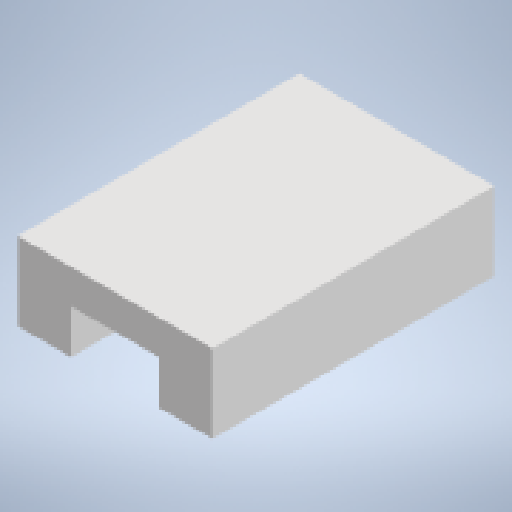
# Autodesk Inventor part: Carrige
Saved by Autodesk Inventor 2023 (Build 270158000, 158)
## iProperties
Created: 2022-09-16
Part Number: Carrige
Material: Generic
Document SubType Name: Modeling
Designer: deli
Density: 1 g/cm^3
Appearance: Default
Author: deli
Autodesk Inventor part; units mm, degrees
ref_plane "YZ Plane" through (0, 0, 0) normal (1, 0, 0) x (0, 1, 0)
ref_plane "XZ Plane" through (0, 0, 0) normal (0, 1, 0) x (-1, 0, 0)
ref_plane "XY Plane" through (0, 0, 0) normal (0, 0, 1) x (1, 0, 0)
sketch "Sketch1" plane through (0, 0, 0) normal (0, 0, 1) x (1, 0, 0)
  line L0 (7.6137, -9.2906) -> (16.6137, -9.2906)
  line L1 (16.6137, -9.2906) -> (16.6137, -13.7906)
  line L2 (7.6137, -13.7906) -> (7.6137, -9.2906)
  line L3 (7.6137, -13.7906) -> (2.1137, -13.7906)
  line L4 (2.1137, -13.7906) -> (2.1137, -5.7906)
  line L5 (2.1137, -5.7906) -> (22.1137, -5.7906)
  line L6 (22.1137, -5.7906) -> (22.1137, -13.7906)
  line L7 (22.1137, -13.7906) -> (16.6137, -13.7906)
  point P0 (0, 0)
  dimension "d0" = 9
  dimension "d1" = 4.5
  dimension "d2" = 4.5
  dimension "d3" = 8
  dimension "d4" = 5.5
  dimension "d5" = 5.5
  constraints: 16 end point, 4 perpendicular, 2 horizontal, 1 parallel, 1 point on line
  measures "d0" distance of L0.start L0.end
  measures "d1" distance of L2.start L0.start
  measures "d2" distance of L0.end L1.end
  measures "d3" distance of L3.end L4.end
  measures "d4" distance of L2.start L3.end
  measures "d5" distance of L6.end L1.end
extrude "Extrusion1" add sketch "Sketch1" along normal blind 28.9
sketch "Sketch2" plane through (2.1137, -5.7906, 0) normal (0, 1, 0) x (1, 0, 0)
  line L0 (20, 0) -> (0, 0) projected
  line L1 (0, 0) -> (0, -28.9) projected
  line L2 (20, -28.9) -> (0, -28.9) projected
  line L3 (20, 0) -> (20, -28.9) projected
  circle A0 centre (17.5, -9.45) radius 1.325
  circle A1 centre (17.5, -19.45) radius 1.325
  circle A2 centre (2.5, -9.45) radius 1.325
  circle A3 centre (2.5, -19.45) radius 1.325
  point P0 (-2.1137, 0)
  dimension "d8" = 2.65
  dimension "d9" = 2.65
  dimension "d10" = 2.65
  dimension "d11" = 2.65
  dimension "d12" = 15
  dimension "d13" = 2.5
  dimension "d14" = 15
  dimension "d15" = 2.5
  dimension "d16" = 10
  dimension "d17" = 9.45
  dimension "d18" = 28.9
  dimension "d19" = 9.45
  dimension "d20" = 10
  constraints: 4 centre point
  measures "d8" diameter of A0
  measures "d9" diameter of A2
  measures "d10" diameter of A3
  measures "d11" diameter of A1
  measures "d12" distance of A2.centre A0.centre
  measures "d13" distance from line of L3 A0.centre
  measures "d14" distance of A3.centre A1.centre
  measures "d15" distance from line of L3 A1.centre
  measures "d16" distance of A1.centre A0.centre
  measures "d17" distance from line of L0 A0.centre
  measures "d18" distance of L0.start L2.start
  measures "d19" distance from line of L0 A2.centre
  measures "d20" distance of A3.centre A2.centre
extrude "Extrusion2" cut sketch "Sketch2" against normal blind 5 contours A0 | A1 | A2 | A3
thread "Thread1" size "M3x0.5" class "6H" standard "ANSI Metric M Profile" full length
thread "Thread2" size "M3x0.5" class "6H" standard "ANSI Metric M Profile" full length
thread "Thread3" size "M3x0.5" class "6H" standard "ANSI Metric M Profile" full length
thread "Thread4" size "M3x0.5" class "6H" standard "ANSI Metric M Profile" full length
sketch "Sketch3" plane through (2.1137, -5.7906, 0) normal (0, 1, 0) x (1, 0, 0)
  line L0 (20, 0) -> (20, -28.9) projected
  line L1 (0, 0) -> (0, -28.9) projected
  line L2 (20, -5) -> (0, -5)
  line L3 (0, -5) -> (0, -23.9)
  line L4 (0, -23.9) -> (20, -23.9)
  line L5 (20, -23.9) -> (20, -5)
  line L6 (20, 0) -> (0, 0) projected
  line L7 (20, -28.9) -> (0, -28.9) projected
  point P0 (-2.1137, 0)
  point P1 (0, -5)
  dimension "d31" = 18.9
  dimension "d32" = 28.9
  dimension "d33" = 5
  constraints: 8 end point, 2 parallel, 2 point on line, 1 horizontal, 1 perpendicular
  measures "d31" distance between parallel lines of L4 L2
  measures "d32" distance of L0.start L0.end
  measures "d33" distance between parallel lines of L6 L2
extrude "Extrusion3" cut sketch "Sketch3" against normal blind 0.5 contours L0 L2 L1 L6 | L0 L7 L1 L4
equation "\"d2\" = d1"
equation "\"d5\" = d4"
equation "\"d9\" = d8"
equation "\"d10\" = d8"
equation "\"d11\" = d8"
equation "\"d14\" = d12"
equation "\"d15\" = d13"
equation "\"d17\" = -0.5 * d16 + 0.5 * d18"
equation "\"d19\" = d17"
equation "\"d20\" = d16"
equation "\"d33\" = -0.5 * d31 + 0.5 * d32"
body "Solid1"
